Autodesk Fusion 360 part; units mm, degrees
(part 2 of 2)
  arc A446 (-3.2604, -44.4999) -> (-4.3604, -44.4999) centre (-3.8104, -44.4999) ccw
  arc A447 (-4.3604, -44.4999) -> (-3.2604, -44.4999) centre (-3.8104, -44.4999) ccw
  arc A448 (-1.8204, -44.4999) -> (-0.7204, -44.4999) centre (-1.2704, -44.4999) ccw
  arc A449 (-0.7204, -44.4999) -> (-1.8204, -44.4999) centre (-1.2704, -44.4999) ccw
  arc A450 (0.7196, -44.4999) -> (1.8196, -44.4999) centre (1.2696, -44.4999) ccw
  arc A451 (1.8196, -44.4999) -> (0.7196, -44.4999) centre (1.2696, -44.4999) ccw
  arc A452 (3.2596, -44.4999) -> (4.3596, -44.4999) centre (3.8096, -44.4999) ccw
  arc A453 (4.3596, -44.4999) -> (3.2596, -44.4999) centre (3.8096, -44.4999) ccw
  arc A454 (6.8996, -44.4999) -> (5.7996, -44.4999) centre (6.3496, -44.4999) ccw
  arc A455 (5.7996, -44.4999) -> (6.8996, -44.4999) centre (6.3496, -44.4999) ccw
  arc A456 (9.4397, -44.4999) -> (8.3396, -44.4999) centre (8.8896, -44.4999) ccw
  arc A457 (8.3396, -44.4999) -> (9.4397, -44.4999) centre (8.8896, -44.4999) ccw
  arc A458 (-8.3404, -88.9997) -> (-9.4404, -88.9997) centre (-8.8904, -88.9997) ccw
  arc A459 (-9.4404, -88.9997) -> (-8.3404, -88.9997) centre (-8.8904, -88.9997) ccw
  arc A460 (-6.9004, -88.9997) -> (-5.8004, -88.9997) centre (-6.3504, -88.9997) ccw
  arc A461 (-5.8004, -88.9997) -> (-6.9004, -88.9997) centre (-6.3504, -88.9997) ccw
  arc A462 (-3.2604, -88.9997) -> (-4.3604, -88.9997) centre (-3.8104, -88.9997) ccw
  arc A463 (-4.3604, -88.9997) -> (-3.2604, -88.9997) centre (-3.8104, -88.9997) ccw
  arc A464 (-0.7204, -88.9997) -> (-1.8204, -88.9997) centre (-1.2704, -88.9997) ccw
  arc A465 (-1.8204, -88.9997) -> (-0.7204, -88.9997) centre (-1.2704, -88.9997) ccw
  arc A466 (1.8196, -88.9997) -> (0.7196, -88.9997) centre (1.2696, -88.9997) ccw
  arc A467 (0.7196, -88.9997) -> (1.8196, -88.9997) centre (1.2696, -88.9997) ccw
  arc A468 (3.2596, -88.9997) -> (4.3596, -88.9997) centre (3.8096, -88.9997) ccw
  arc A469 (4.3596, -88.9997) -> (3.2596, -88.9997) centre (3.8096, -88.9997) ccw
  arc A470 (5.7996, -88.9997) -> (6.8996, -88.9997) centre (6.3496, -88.9997) ccw
  arc A471 (6.8996, -88.9997) -> (5.7996, -88.9997) centre (6.3496, -88.9997) ccw
  arc A472 (8.3396, -88.9997) -> (9.4397, -88.9997) centre (8.8896, -88.9997) ccw
  arc A473 (9.4397, -88.9997) -> (8.3396, -88.9997) centre (8.8896, -88.9997) ccw
  arc A474 (-0.3229, -73.4261) -> (0.5771, -73.4261) centre (0.1271, -73.4261) ccw
  arc A475 (0.5771, -73.4261) -> (-0.3229, -73.4261) centre (0.1271, -73.4261) ccw
  arc A476 (0.5771, -75.9261) -> (-0.3229, -75.9261) centre (0.1271, -75.9261) ccw
  arc A477 (-0.3229, -75.9261) -> (0.5771, -75.9261) centre (0.1271, -75.9261) ccw
  arc A478 (5.8685, -67.4771) -> (5.5635, -67.4771) centre (5.716, -67.4771) ccw
  arc A479 (5.5635, -67.4771) -> (5.8685, -67.4771) centre (5.716, -67.4771) ccw
  arc A480 (4.0575, -72.148) -> (3.7525, -72.148) centre (3.905, -72.148) ccw
  arc A481 (3.7525, -72.148) -> (4.0575, -72.148) centre (3.905, -72.148) ccw
  circle A482 centre (15, -5) radius 1
  dimension "d42" = 2
  dimension "d43" = 4.9999
  dimension "d44" = 15
  measures "d42" diameter of A482
  measures "d43" vertical distance of A420.end A482.centre
  measures "d44" horizontal distance of origin A482.centre
extrude "Extrude6" add sketch "DXF_PCB3_2026-08-19_AutoCAD2007" along normal blind 1.6 separate body contours L0 A0 A1 L1 A2 L2 L3 A3 | A482 makes body 2
move_body "Move1" bodies 2 to x (1, 0, 0) y (0, 1, 0) z (0, 0, 1) at (1.5, 103, 21.6)
move_body "Move2" bodies 2 to x (1, 0, 0) y (0, 1, 0) z (0, 0, 1) at (0, 7, 0)
sketch "Sketch4" plane through (0, -27, 0) normal (0, 1, 0) x (-1, 0, 0)
  line L0 (-333.5, 5) -> (22, 5)
  line L1 (22, 40) -> (-333.5, 40)
  circle A0 centre (18, 40) radius 4
  line L2 (22, 5) -> (22, 40)
  line L3 (-333.5, 40) -> (-333.5, 5)
  constraint coincident L1 A0.centre
extrude "Extrude7" cut sketch "Sketch4" against normal blind 2.3 contours L1 A0 picked at (16.6816, 39.8013) bodies 1
sketch "Sketch5" plane through (-24, 0, 0) normal (1, 0, 0) x (0, 1, 0)
  line L0 (-25, 5) -> (114, 5)
  circle A0 centre (-21, 40) radius 4
  line L1 (114, 5) -> (114, 40)
  line L2 (114, 40) -> (-25, 40)
  line L3 (-25, 40) -> (-25, 5)
extrude "Extrude8" cut sketch "Sketch5" against normal blind 2.3 contours A0 L2 picked at (-19.6816, 39.8013) bodies 1
move_body "Move3" bodies 2 to x (1, 0, 0) y (0, 1, 0) z (0, 0, 1) at (-1.5, 0, 0)
fillet "Fillet2" radius 1.2 32 edges at (155.75, -30, 0) (337.0355, -28.5355, 0) (338.5, 44.5, 0) (337.0355, 117.5355, 0) (155.75, 119, 0) (-25.5355, 117.5355, 0) (-27, 44.5, 0) (-25.5355, -28.5355, 0) (-15.0105, 50.322, 0) (-15.0105, 5.822, 0) (-15.0105, 94.822, 0) (29.4895, 50.322, 0) (29.4895, 5.822, 0) (29.4895, 94.822, 0) (73.9895, 50.322, 0) (73.9895, 5.822, 0) (118.4895, 5.822, 0) (118.4895, 50.322, 0) (162.9895, 5.822, 0) (162.9895, 50.322, 0) (207.4895, 5.822, 0) (251.9895, 5.822, 0) (207.4895, 50.322, 0) (162.9895, 94.822, 0) (118.4895, 94.822, 0) (73.9895, 94.822, 0) (251.9895, 50.322, 0) (296.4895, 5.822, 0) (207.4895, 94.822, 0) (251.9895, 94.822, 0) (296.4895, 50.322, 0) (296.4895, 94.822, 0) on bodies 1
ref_plane "WorkPlane1" through (156, 44.5, 20.6) normal (-1, 0, 0) x (0, -1, 0)
split "Split1" [rolled back]
sketch "Sketch6" plane through (156, 0, 0) normal (1, 0, 0) x (0, 1, 0)
  line L0 (116, 5) -> (-27, 5)
  line L1 (-27, 5) -> (-27, 40)
  line L2 (-27, 40) -> (-30, 40)
  line L3 (-30, 40) -> (-30, 1.2)
  arc A0 (-30, 1.2) -> (-28.8, 0) centre (-28.8, 1.2) ccw
  line L4 (-28.8, 0) -> (117.8, 0)
  arc A1 (117.8, 0) -> (119, 1.2) centre (117.8, 1.2) ccw
  line L5 (119, 1.2) -> (119, 40)
  line L6 (119, 40) -> (116, 40)
  line L7 (116, 40) -> (116, 5)
  circle A2 centre (-21, 2.5) radius 0.975
  circle A3 centre (22.6667, 2.5) radius 0.975
  circle A4 centre (66.3333, 2.5) radius 0.975
  circle A5 centre (110, 2.5) radius 0.975
  circle A6 centre (117.5, 35.5) radius 0.9975
  circle A7 centre (-28.5, 35.5) radius 0.9975
  circle A8 centre (117.5, 12.5) radius 0.9975
  circle A9 centre (-28.5, 12.5) radius 0.9975
  dimension "d49" = 1.95
  dimension "d52" = 131
  dimension "d53" = 0
  dimension "d58" = 1.995
  dimension "d61" = -146
  dimension "d62" = -23
  measures "d49" diameter of A2
  measures "d58" diameter of A6
extrude "Extrude10" [rolled back] along distance -20 taper angle 0
extrude "Extrude9" [rolled back] along distance 20 taper angle 0
combine "Combine2" [rolled back]
hidden bodies 2
equation "d14 = ( 44.5 * 7 ) * 1 mm"
equation "d15 = dist * 2"
equation "dist = 44.5 mm"
equation "d17 = dist_b - 2 mm"
equation "d18 = dist_b - 2 mm"
equation "d19 = dist_b + 1 mm"
equation "d20 = dist_b + 1 mm"
equation "dist_b = 29 mm"
equation "d47 = ( -365.00 / 2 ) * 1 mm - 0.5 mm"
named bodies: "ClockClock24", "ClockClock24 (1)"
